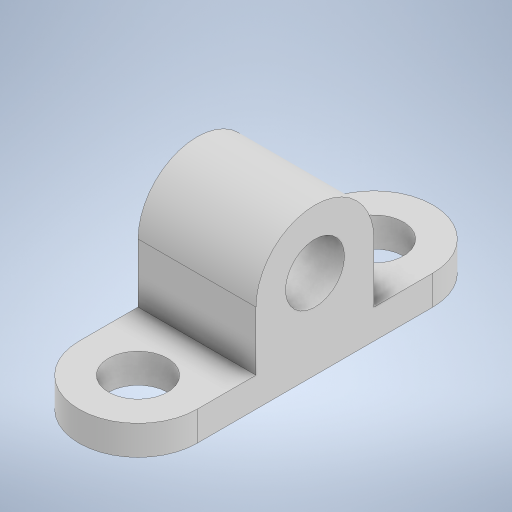
# Autodesk Inventor part: Actividad#1
Saved by Autodesk Inventor 2024 (Build 280153000, 153)
## iProperties
Created: 2024-02-04
Part Number: Actividad#1
Material: Genérico
Document SubType Name: Modeling
Designer: 50254
Density: 1 g/cm^3
Appearance: Valor por defecto
Author: 50254
Autodesk Inventor part; units mm, degrees
ref_plane "YZ Plane" through (0, 0, 0) normal (1, 0, 0) x (0, 1, 0)
ref_plane "XZ Plane" through (0, 0, 0) normal (0, 1, 0) x (-1, 0, 0)
ref_plane "XY Plane" through (0, 0, 0) normal (0, 0, 1) x (1, 0, 0)
sketch "Boceto1" plane through (0, 0, 0) normal (0, 1, 0) x (-1, 0, 0)
  line L0 (20, -20) -> (20, 20)
  line L1 (-20, 20) -> (-20, -20)
  line L2 (-20, -20) -> (20, 20) construction
  line L3 (20, -20) -> (-20, 20) construction
  line L4 (0, 20) -> (0, 40) construction
  circle A0 centre (0, 40) radius 10
  arc A1 (20, 40) -> (-20, 40) centre (0, 40) ccw
  line L5 (0, -20) -> (0, -40) construction
  circle A2 centre (0, -40) radius 10
  arc A3 (-20, -40) -> (20, -40) centre (0, -40) ccw
  line L6 (20, 40) -> (20, 20)
  line L7 (-20, 40) -> (-20, 20)
  line L8 (20, -40) -> (20, -20)
  line L9 (-20, -20) -> (-20, -40)
  point P0 (0, 0)
  dimension "d1" = 40
  dimension "d3" = 20
  dimension "d4" = 40
  dimension "d6" = 20
  dimension "d7" = 40
  constraints: 20 end point, 4 centre point, 4 coincident, 4 point on circle, 3 vertical, 2 midpoint, 2 tangent, 1 parallel, 1 point on line
  measures "d1" distance of L0.end L0.start
  measures "d3" diameter of A0
  measures "d4" diameter of A1
  measures "d6" diameter of A2
  measures "d7" diameter of A3
extrude "Extrusión1" add sketch "Boceto1" along normal blind 10
sketch "Boceto2" plane through (20, 0, 40) normal (1, 0, 0) x (0, 0, -1)
  line L0 (0, 10) -> (80, 10) construction
  line L1 (40, 10) -> (40, 30) construction
  line L2 (40, 10) -> (60, 10) construction
  arc A0 (60, 30) -> (20, 30) centre (40, 30) ccw
  circle A1 centre (40, 30) radius 10
  line L3 (20, 30) -> (20, 10)
  line L4 (60, 30) -> (60, 10)
  line L5 (20, 10) -> (60, 10)
  point P0 (40, 0)
  dimension "d12" = 40
  dimension "d13" = 20
  constraints: 10 end point, 3 perpendicular, 2 centre point, 2 coincident, 2 midpoint, 2 point on circle, 2 tangent, 1 collinear, 1 horizontal, 1 point on line, 1 vertical
  measures "d12" diameter of A0
  measures "d13" diameter of A1
extrude "Extrusión2" add sketch "Boceto2" against normal blind 40
